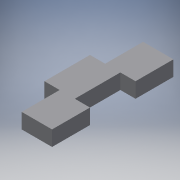
# Autodesk Inventor part: Part14
Saved by Autodesk Inventor 2018 (Build 220112000, 112)
## iProperties
Created: 2018-05-23
Part Number: Part14
Material: Generic
Document SubType Name: Modeling
Designer: lenovo
Density: 1 g/cm^3
Appearance: Default
Author: lenovo
Autodesk Inventor part; units mm, degrees
ref_plane "YZ Plane" through (0, 0, 0) normal (1, 0, 0) x (0, 1, 0)
ref_plane "XZ Plane" through (0, 0, 0) normal (0, 1, 0) x (-1, 0, 0)
ref_plane "XY Plane" through (0, 0, 0) normal (0, 0, 1) x (1, 0, 0)
sketch "Sketch1" plane through (0, 0, 0) normal (0, 1, 0) x (-1, 0, 0)
  line L0 (-25.4, 49.2125) -> (-31.75, 49.2125)
  line L1 (-31.75, 49.2125) -> (-31.75, 23.8125)
  line L2 (-31.75, 23.8125) -> (-25.4, 23.8125)
  line L3 (-25.4, 23.8125) -> (-25.4, 49.2125)
  line L4 (-25.4, 41.275) -> (-22.225, 41.275)
  line L5 (-22.225, 41.275) -> (-22.225, 31.75)
  line L6 (-22.225, 31.75) -> (-25.4, 31.75)
  line L7 (-25.4, 31.75) -> (-25.4, 41.275)
  line L8 (-31.75, 41.275) -> (-28.575, 41.275)
  line L9 (-28.575, 41.275) -> (-28.575, 31.75)
  line L10 (-28.575, 31.75) -> (-31.75, 31.75)
  line L11 (-31.75, 31.75) -> (-31.75, 41.275)
  point P0 (0, 0)
  dimension "d0" = 7.9375
  dimension "d1" = 7.9375
  dimension "d2" = 25.4
  dimension "d3" = 3.175
  dimension "d4" = 6.35
  dimension "d5" = 3.175
  constraints: 24 end point, 6 parallel, 4 point on line, 3 horizontal, 3 perpendicular
  measures "d0" distance between parallel lines of L0 L4
  measures "d1" distance between parallel lines of L2 L6
  measures "d2" distance between parallel lines of L2 L0
  measures "d3" distance between parallel lines of L5 L3
  measures "d4" distance between parallel lines of L1 L3
  measures "d5" distance between parallel lines of L1 L9
extrude "Extrusion1" add sketch "Sketch1" along normal blind 3.175 contours L3 L2 L1 L10 L9 L8 L0 | L4 L5 L6 L3
body "Solid1"
